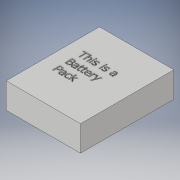
# Autodesk Inventor part: DPLX_P018_Crude_Battery_Placeholder_Smalltestmod
Saved by Autodesk Inventor 2018 (Build 220112000, 112)
## iProperties
Created: 2018-06-13
Part Number: DPLX_P018_Crude_Battery_Placeholder_Smalltestmod
Material: Generic
Document SubType Name: Modeling
Designer: DPLXuser
Density: 1 g/cm^3
Appearance: Default
Author: DPLXuser
Autodesk Inventor part; units mm, degrees
ref_plane "YZ Plane" through (0, 0, 0) normal (1, 0, 0) x (0, 1, 0)
ref_plane "XZ Plane" through (0, 0, 0) normal (0, 1, 0) x (-1, 0, 0)
ref_plane "XY Plane" through (0, 0, 0) normal (0, 0, 1) x (1, 0, 0)
sketch "Sketch1" plane through (0, 0, 0) normal (0, 1, 0) x (-1, 0, 0)
  line L0 (-30.353, 38.1) -> (30.353, 38.1)
  line L1 (30.353, 38.1) -> (30.353, -38.1)
  line L2 (30.353, -38.1) -> (-30.353, -38.1)
  line L3 (-30.353, -38.1) -> (-30.353, 38.1)
  line L4 (-30.353, 38.1) -> (30.353, -38.1) construction
  line L5 (30.353, 38.1) -> (-30.353, -38.1) construction
  point P0 (0, 0)
  dimension "d0" = 60.706
  dimension "d1" = 76.2
  constraints: 12 end point, 2 midpoint, 2 parallel, 1 horizontal, 1 perpendicular
  measures "d0" distance of L1.end L2.end
  measures "d1" distance of L0.end L1.end
extrude "Extrusion1" add sketch "Sketch1" along normal blind 20.828
sketch "Sketch2" plane through (0, 20.828, 0) normal (0, 1, 0) x (1, 0, 0)
  line L0 (-19.6689, 24.4409) -> (19.4476, 24.4409) construction
  line L1 (19.4476, 24.4409) -> (19.4476, -21.2872) construction
  line L2 (19.4476, -21.2872) -> (-19.6689, -21.2872) construction
  line L3 (-19.6689, -21.2872) -> (-19.6689, 24.4409) construction
  line L4 (-17.6287, 8.4941) -> (-17.6287, 13.8689)
  line L5 (-17.6287, 13.8689) -> (-19.6739, 13.8689)
  line L6 (-19.6739, 13.8689) -> (-19.6739, 14.5901)
  line L7 (-19.6739, 14.5901) -> (-14.7734, 14.5901)
  line L8 (-14.7734, 14.5901) -> (-14.7734, 13.8689)
  line L9 (-14.7734, 13.8689) -> (-16.8185, 13.8689)
  line L10 (-16.8185, 13.8689) -> (-16.8185, 8.4941)
  line L11 (-16.8185, 8.4941) -> (-17.6287, 8.4941)
  line L12 (-10.6237, 8.4941) -> (-11.3944, 8.4941)
  line L13 (-11.3944, 8.4941) -> (-11.3944, 11.1024)
  spline S0 degree 2 poles (-11.3944, 11.1024) (-11.3944, 11.4186) (-11.4537, 11.962) (-11.5426, 12.125) knots 0 0 0 1 2 2 2
  spline S1 degree 2 poles (-11.5426, 12.125) (-11.6364, 12.2979) (-11.9724, 12.4659) (-12.2589, 12.4659) knots 0 0 0 1 2 2 2
  spline S2 degree 2 poles (-12.2589, 12.4659) (-12.5454, 12.4659) (-13.153, 12.1596) (-13.4445, 11.9126) knots 0 0 0 1 2 2 2
  line L14 (-13.4445, 11.9126) -> (-13.4445, 8.4941)
  line L15 (-13.4445, 8.4941) -> (-14.2151, 8.4941)
  line L16 (-14.2151, 8.4941) -> (-14.2151, 14.8618)
  line L17 (-14.2151, 14.8618) -> (-13.4445, 14.8618)
  line L18 (-13.4445, 14.8618) -> (-13.4445, 12.5598)
  spline S3 degree 2 poles (-13.4445, 12.5598) (-13.0987, 12.871) (-12.4318, 13.197) (-12.0563, 13.197) knots 0 0 0 1 2 2 2
  spline S4 degree 2 poles (-12.0563, 13.197) (-11.3845, 13.197) (-10.6237, 12.3078) (-10.6237, 11.4631) knots 0 0 0 1 2 2 2
  line L19 (-10.6237, 11.4631) -> (-10.6237, 8.4941)
  line L20 (-8.7564, 8.4941) -> (-9.527, 8.4941)
  line L21 (-9.527, 8.4941) -> (-9.527, 13.0686)
  line L22 (-9.527, 13.0686) -> (-8.7564, 13.0686)
  line L23 (-8.7564, 13.0686) -> (-8.7564, 8.4941)
  line L24 (-8.7021, 13.8293) -> (-9.5764, 13.8293)
  line L25 (-9.5764, 13.8293) -> (-9.5764, 14.6296)
  line L26 (-9.5764, 14.6296) -> (-8.7021, 14.6296)
  line L27 (-8.7021, 14.6296) -> (-8.7021, 13.8293)
  spline S5 degree 2 poles (-6.3901, 8.3854) (-6.8495, 8.3854) (-7.6449, 8.6324) (-7.9067, 8.7707) knots 0 0 0 1 2 2 2
  line L28 (-7.9067, 8.7707) -> (-7.9067, 9.6353)
  line L29 (-7.9067, 9.6353) -> (-7.8672, 9.6353)
  spline S6 degree 2 poles (-7.8672, 9.6353) (-7.7684, 9.5562) (-7.5016, 9.3685) (-7.2793, 9.2648) knots 0 0 0 1 2 2 2
  spline S7 degree 2 poles (-7.2793, 9.2648) (-7.0867, 9.1709) (-6.6124, 9.0326) (-6.3605, 9.0326) knots 0 0 0 1 2 2 2
  spline S8 degree 2 poles (-6.3605, 9.0326) (-6.1777, 9.0326) (-5.7578, 9.1165) (-5.659, 9.1857) knots 0 0 0 1 2 2 2
  spline S9 degree 2 poles (-5.659, 9.1857) (-5.5157, 9.2796) (-5.3873, 9.492) (-5.3873, 9.7094) knots 0 0 0 1 2 2 2
  spline S10 degree 2 poles (-5.3873, 9.7094) (-5.3873, 9.9811) (-5.6837, 10.2626) (-6.0641, 10.3565) knots 0 0 0 1 2 2 2
  spline S11 degree 2 poles (-6.0641, 10.3565) (-6.2123, 10.3911) (-6.6865, 10.4899) (-6.8891, 10.5442) knots 0 0 0 1 2 2 2
  spline S12 degree 2 poles (-6.8891, 10.5442) (-7.4127, 10.6974) (-7.8869, 11.3297) (-7.8869, 11.7792) knots 0 0 0 1 2 2 2
  spline S13 degree 2 poles (-7.8869, 11.7792) (-7.8869, 12.4017) (-6.9533, 13.1773) (-6.1826, 13.1773) knots 0 0 0 1 2 2 2
  spline S14 degree 2 poles (-6.1826, 13.1773) (-5.8023, 13.1773) (-5.0316, 12.9895) (-4.7698, 12.8463) knots 0 0 0 1 2 2 2
  line L30 (-4.7698, 12.8463) -> (-4.7698, 12.0213)
  line L31 (-4.7698, 12.0213) -> (-4.8093, 12.0213)
  spline S15 degree 2 poles (-4.8093, 12.0213) (-5.1057, 12.2584) (-5.827, 12.5301) (-6.1975, 12.5301) knots 0 0 0 1 2 2 2
  spline S16 degree 2 poles (-6.1975, 12.5301) (-6.5778, 12.5301) (-7.1015, 12.209) (-7.1015, 11.8879) knots 0 0 0 1 2 2 2
  spline S17 degree 2 poles (-7.1015, 11.8879) (-7.1015, 11.5964) (-6.7903, 11.3149) (-6.4445, 11.2259) knots 0 0 0 1 2 2 2
  spline S18 degree 2 poles (-6.4445, 11.2259) (-6.2765, 11.1815) (-5.8517, 11.0926) (-5.6195, 11.0382) knots 0 0 0 1 2 2 2
  spline S19 degree 2 poles (-5.6195, 11.0382) (-5.1156, 10.9098) (-4.6018, 10.3219) (-4.6018, 9.8131) knots 0 0 0 1 2 2 2
  spline S20 degree 2 poles (-4.6018, 9.8131) (-4.6018, 9.5167) (-4.834, 8.993) (-5.0612, 8.8004) knots 0 0 0 1 2 2 2
  spline S21 degree 2 poles (-5.0612, 8.8004) (-5.3033, 8.5978) (-5.9208, 8.3854) (-6.3901, 8.3854) knots 0 0 0 1 2 2 2
  line L32 (-0.4818, 8.4941) -> (-1.2525, 8.4941)
  line L33 (-1.2525, 8.4941) -> (-1.2525, 13.0686)
  line L34 (-1.2525, 13.0686) -> (-0.4818, 13.0686)
  line L35 (-0.4818, 13.0686) -> (-0.4818, 8.4941)
  line L36 (-0.4275, 13.8293) -> (-1.3019, 13.8293)
  line L37 (-1.3019, 13.8293) -> (-1.3019, 14.6296)
  line L38 (-1.3019, 14.6296) -> (-0.4275, 14.6296)
  line L39 (-0.4275, 14.6296) -> (-0.4275, 13.8293)
  spline S22 degree 2 poles (1.8844, 8.3854) (1.425, 8.3854) (0.6297, 8.6324) (0.3678, 8.7707) knots 0 0 0 1 2 2 2
  line L40 (0.3678, 8.7707) -> (0.3678, 9.6353)
  line L41 (0.3678, 9.6353) -> (0.4074, 9.6353)
  spline S23 degree 2 poles (0.4074, 9.6353) (0.5062, 9.5562) (0.7729, 9.3685) (0.9952, 9.2648) knots 0 0 0 1 2 2 2
  spline S24 degree 2 poles (0.9952, 9.2648) (1.1879, 9.1709) (1.6621, 9.0326) (1.9141, 9.0326) knots 0 0 0 1 2 2 2
  spline S25 degree 2 poles (1.9141, 9.0326) (2.0969, 9.0326) (2.5168, 9.1165) (2.6156, 9.1857) knots 0 0 0 1 2 2 2
  spline S26 degree 2 poles (2.6156, 9.1857) (2.7588, 9.2796) (2.8873, 9.492) (2.8873, 9.7094) knots 0 0 0 1 2 2 2
  spline S27 degree 2 poles (2.8873, 9.7094) (2.8873, 9.9811) (2.5909, 10.2626) (2.2105, 10.3565) knots 0 0 0 1 2 2 2
  spline S28 degree 2 poles (2.2105, 10.3565) (2.0623, 10.3911) (1.588, 10.4899) (1.3855, 10.5442) knots 0 0 0 1 2 2 2
  spline S29 degree 2 poles (1.3855, 10.5442) (0.8619, 10.6974) (0.3876, 11.3297) (0.3876, 11.7792) knots 0 0 0 1 2 2 2
  spline S30 degree 2 poles (0.3876, 11.7792) (0.3876, 12.4017) (1.3213, 13.1773) (2.0919, 13.1773) knots 0 0 0 1 2 2 2
  spline S31 degree 2 poles (2.0919, 13.1773) (2.4723, 13.1773) (3.2429, 12.9895) (3.5048, 12.8463) knots 0 0 0 1 2 2 2
  line L42 (3.5048, 12.8463) -> (3.5048, 12.0213)
  line L43 (3.5048, 12.0213) -> (3.4652, 12.0213)
  spline S32 degree 2 poles (3.4652, 12.0213) (3.1688, 12.2584) (2.4476, 12.5301) (2.0771, 12.5301) knots 0 0 0 1 2 2 2
  spline S33 degree 2 poles (2.0771, 12.5301) (1.6967, 12.5301) (1.1731, 12.209) (1.1731, 11.8879) knots 0 0 0 1 2 2 2
  spline S34 degree 2 poles (1.1731, 11.8879) (1.1731, 11.5964) (1.4843, 11.3149) (1.8301, 11.2259) knots 0 0 0 1 2 2 2
  spline S35 degree 2 poles (1.8301, 11.2259) (1.9981, 11.1815) (2.4229, 11.0926) (2.6551, 11.0382) knots 0 0 0 1 2 2 2
  spline S36 degree 2 poles (2.6551, 11.0382) (3.159, 10.9098) (3.6727, 10.3219) (3.6727, 9.8131) knots 0 0 0 1 2 2 2
  spline S37 degree 2 poles (3.6727, 9.8131) (3.6727, 9.5167) (3.4405, 8.993) (3.2133, 8.8004) knots 0 0 0 1 2 2 2
  spline S38 degree 2 poles (3.2133, 8.8004) (2.9712, 8.5978) (2.3537, 8.3854) (1.8844, 8.3854) knots 0 0 0 1 2 2 2
  spline S39 degree 2 poles (9.5563, 8.9782) (9.4624, 8.9091) (9.1463, 8.6621) (8.9981, 8.588) knots 0 0 0 1 2 2 2
  spline S40 degree 2 poles (8.9981, 8.588) (8.7955, 8.4793) (8.4152, 8.3657) (8.0694, 8.3657) knots 0 0 0 1 2 2 2
  spline S41 degree 2 poles (8.0694, 8.3657) (7.7878, 8.3657) (7.279, 8.5781) (7.0863, 8.7707) knots 0 0 0 1 2 2 2
  spline S42 degree 2 poles (7.0863, 8.7707) (6.9035, 8.9585) (6.6812, 9.5118) (6.6812, 9.818) knots 0 0 0 1 2 2 2
  spline S43 degree 2 poles (6.6812, 9.818) (6.6812, 10.2923) (7.0814, 10.9641) (7.5161, 11.1568) knots 0 0 0 1 2 2 2
  spline S44 degree 2 poles (7.5161, 11.1568) (7.9014, 11.3346) (8.9487, 11.468) (9.5563, 11.5026) knots 0 0 0 1 2 2 2
  line L44 (9.5563, 11.5026) -> (9.5563, 11.6508)
  spline S45 degree 2 poles (9.5563, 11.6508) (9.5563, 11.9175) (9.3933, 12.2485) (9.2451, 12.3424) knots 0 0 0 1 2 2 2
  spline S46 degree 2 poles (9.2451, 12.3424) (9.0969, 12.4363) (8.672, 12.4955) (8.4448, 12.4955) knots 0 0 0 1 2 2 2
  spline S47 degree 2 poles (8.4448, 12.4955) (8.178, 12.4955) (7.4568, 12.3375) (7.0962, 12.1843) knots 0 0 0 1 2 2 2
  line L45 (7.0962, 12.1843) -> (7.0517, 12.1843)
  line L46 (7.0517, 12.1843) -> (7.0517, 12.9698)
  spline S48 degree 2 poles (7.0517, 12.9698) (7.2641, 13.0291) (8.0595, 13.1773) (8.4497, 13.1773) knots 0 0 0 1 2 2 2
  spline S49 degree 2 poles (8.4497, 13.1773) (8.924, 13.1773) (9.5711, 13.0291) (9.828, 12.8364) knots 0 0 0 1 2 2 2
  spline S50 degree 2 poles (9.828, 12.8364) (10.08, 12.6487) (10.327, 12.0509) (10.327, 11.6211) knots 0 0 0 1 2 2 2
  line L47 (10.327, 11.6211) -> (10.327, 8.4941)
  line L48 (10.327, 8.4941) -> (9.5563, 8.4941)
  line L49 (9.5563, 8.4941) -> (9.5563, 8.9782)
  line L50 (9.5563, 9.6204) -> (9.5563, 10.89)
  spline S51 degree 2 poles (9.5563, 10.89) (9.2797, 10.8653) (8.4448, 10.7813) (8.183, 10.7023) knots 0 0 0 1 2 2 2
  spline S52 degree 2 poles (8.183, 10.7023) (7.8767, 10.6084) (7.4766, 10.2182) (7.4766, 9.8724) knots 0 0 0 1 2 2 2
  spline S53 degree 2 poles (7.4766, 9.8724) (7.4766, 9.4772) (7.9212, 9.077) (8.346, 9.077) knots 0 0 0 1 2 2 2
  spline S54 degree 2 poles (8.346, 9.077) (8.7066, 9.077) (9.2994, 9.3883) (9.5563, 9.6204) knots 0 0 0 1 2 2 2
  spline S55 degree 2 poles (-14.9166, 0.3295) (-14.9166, -0.125) (-15.2624, -0.8216) (-15.5489, -1.0488) knots 0 0 0 1 2 2 2
  spline S56 degree 2 poles (-15.5489, -1.0488) (-15.8947, -1.3156) (-16.6802, -1.5428) (-17.3026, -1.5428) knots 0 0 0 1 2 2 2
  line L51 (-17.3026, -1.5428) -> (-19.0514, -1.5428)
  line L52 (-19.0514, -1.5428) -> (-19.0514, 4.5532)
  line L53 (-19.0514, 4.5532) -> (-17.436, 4.5532)
  spline S57 degree 2 poles (-17.436, 4.5532) (-16.7839, 4.5532) (-16.1319, 4.4692) (-15.8355, 4.3062) knots 0 0 0 1 2 2 2
  spline S58 degree 2 poles (-15.8355, 4.3062) (-15.5045, 4.1333) (-15.2031, 3.5652) (-15.2031, 3.1799) knots 0 0 0 1 2 2 2
  spline S59 degree 2 poles (-15.2031, 3.1799) (-15.2031, 2.7501) (-15.6576, 2.0684) (-16.0578, 1.8757) knots 0 0 0 1 2 2 2
  line L54 (-16.0578, 1.8757) -> (-16.0578, 1.8461)
  spline S60 degree 2 poles (-16.0578, 1.8461) (-15.5144, 1.6979) (-14.9166, 0.9124) (-14.9166, 0.3295) knots 0 0 0 1 2 2 2
  spline S61 degree 2 poles (-15.7614, 0.2949) (-15.7614, 0.6407) (-15.959, 1.0853) (-16.2554, 1.2434) knots 0 0 0 1 2 2 2
  spline S62 degree 2 poles (-16.2554, 1.2434) (-16.448, 1.3422) (-16.9025, 1.4015) (-17.3224, 1.4015) knots 0 0 0 1 2 2 2
  line L55 (-17.3224, 1.4015) -> (-18.2413, 1.4015)
  line L56 (-18.2413, 1.4015) -> (-18.2413, -0.8512)
  line L57 (-18.2413, -0.8512) -> (-17.5842, -0.8512)
  spline S63 degree 2 poles (-17.5842, -0.8512) (-17.0507, -0.8512) (-16.4381, -0.7524) (-16.201, -0.5943) knots 0 0 0 1 2 2 2
  spline S64 degree 2 poles (-16.201, -0.5943) (-15.9738, -0.4313) (-15.7614, -0.0262) (-15.7614, 0.2949) knots 0 0 0 1 2 2 2
  spline S65 degree 2 poles (-16.0479, 3.0663) (-16.0479, 3.2836) (-16.1961, 3.6097) (-16.3591, 3.7035) knots 0 0 0 1 2 2 2
  spline S66 degree 2 poles (-16.3591, 3.7035) (-16.5567, 3.8122) (-17.0359, 3.8616) (-17.4657, 3.8616) knots 0 0 0 1 2 2 2
  line L58 (-17.4657, 3.8616) -> (-18.2413, 3.8616)
  line L59 (-18.2413, 3.8616) -> (-18.2413, 2.0782)
  line L60 (-18.2413, 2.0782) -> (-17.3224, 2.0782)
  spline S67 degree 2 poles (-17.3224, 2.0782) (-16.942, 2.0782) (-16.5814, 2.1573) (-16.3887, 2.2808) knots 0 0 0 1 2 2 2
  spline S68 degree 2 poles (-16.3887, 2.2808) (-16.201, 2.3993) (-16.0479, 2.7797) (-16.0479, 3.0663) knots 0 0 0 1 2 2 2
  spline S69 degree 2 poles (-11.6216, -1.0587) (-11.7155, -1.1278) (-12.0316, -1.3748) (-12.1798, -1.4489) knots 0 0 0 1 2 2 2
  spline S70 degree 2 poles (-12.1798, -1.4489) (-12.3824, -1.5576) (-12.7628, -1.6712) (-13.1086, -1.6712) knots 0 0 0 1 2 2 2
  spline S71 degree 2 poles (-13.1086, -1.6712) (-13.3901, -1.6712) (-13.899, -1.4588) (-14.0916, -1.2662) knots 0 0 0 1 2 2 2
  spline S72 degree 2 poles (-14.0916, -1.2662) (-14.2744, -1.0784) (-14.4967, -0.5252) (-14.4967, -0.2189) knots 0 0 0 1 2 2 2
  spline S73 degree 2 poles (-14.4967, -0.2189) (-14.4967, 0.2554) (-14.0966, 0.9272) (-13.6618, 1.1199) knots 0 0 0 1 2 2 2
  spline S74 degree 2 poles (-13.6618, 1.1199) (-13.2765, 1.2977) (-12.2292, 1.4311) (-11.6216, 1.4657) knots 0 0 0 1 2 2 2
  line L61 (-11.6216, 1.4657) -> (-11.6216, 1.6139)
  spline S75 degree 2 poles (-11.6216, 1.6139) (-11.6216, 1.8806) (-11.7846, 2.2116) (-11.9328, 2.3055) knots 0 0 0 1 2 2 2
  spline S76 degree 2 poles (-11.9328, 2.3055) (-12.081, 2.3993) (-12.5059, 2.4586) (-12.7331, 2.4586) knots 0 0 0 1 2 2 2
  spline S77 degree 2 poles (-12.7331, 2.4586) (-12.9999, 2.4586) (-13.7211, 2.3005) (-14.0817, 2.1474) knots 0 0 0 1 2 2 2
  line L62 (-14.0817, 2.1474) -> (-14.1262, 2.1474)
  line L63 (-14.1262, 2.1474) -> (-14.1262, 2.9329)
  spline S78 degree 2 poles (-14.1262, 2.9329) (-13.9138, 2.9922) (-13.1184, 3.1404) (-12.7282, 3.1404) knots 0 0 0 1 2 2 2
  spline S79 degree 2 poles (-12.7282, 3.1404) (-12.2539, 3.1404) (-11.6068, 2.9922) (-11.3499, 2.7995) knots 0 0 0 1 2 2 2
  spline S80 degree 2 poles (-11.3499, 2.7995) (-11.098, 2.6118) (-10.851, 2.014) (-10.851, 1.5842) knots 0 0 0 1 2 2 2
  line L64 (-10.851, 1.5842) -> (-10.851, -1.5428)
  line L65 (-10.851, -1.5428) -> (-11.6216, -1.5428)
  line L66 (-11.6216, -1.5428) -> (-11.6216, -1.0587)
  line L67 (-11.6216, -0.4165) -> (-11.6216, 0.8531)
  spline S81 degree 2 poles (-11.6216, 0.8531) (-11.8983, 0.8284) (-12.7331, 0.7444) (-12.9949, 0.6654) knots 0 0 0 1 2 2 2
  spline S82 degree 2 poles (-12.9949, 0.6654) (-13.3012, 0.5715) (-13.7014, 0.1813) (-13.7014, -0.1645) knots 0 0 0 1 2 2 2
  spline S83 degree 2 poles (-13.7014, -0.1645) (-13.7014, -0.5597) (-13.2568, -0.9599) (-12.8319, -0.9599) knots 0 0 0 1 2 2 2
  spline S84 degree 2 poles (-12.8319, -0.9599) (-12.4713, -0.9599) (-11.8785, -0.6487) (-11.6216, -0.4165) knots 0 0 0 1 2 2 2
  spline S85 degree 2 poles (-8.3859, -1.6317) (-9.0133, -1.6317) (-9.7197, -0.9154) (-9.7197, -0.1398) knots 0 0 0 1 2 2 2
  line L68 (-9.7197, -0.1398) -> (-9.7197, 2.3944)
  line L69 (-9.7197, 2.3944) -> (-10.2384, 2.3944)
  line L70 (-10.2384, 2.3944) -> (-10.2384, 3.0317)
  line L71 (-10.2384, 3.0317) -> (-9.7197, 3.0317)
  line L72 (-9.7197, 3.0317) -> (-9.7197, 4.3457)
  line L73 (-9.7197, 4.3457) -> (-8.9491, 4.3457)
  line L74 (-8.9491, 4.3457) -> (-8.9491, 3.0317)
  line L75 (-8.9491, 3.0317) -> (-7.5313, 3.0317)
  line L76 (-7.5313, 3.0317) -> (-7.5313, 2.3944)
  line L77 (-7.5313, 2.3944) -> (-8.9491, 2.3944)
  line L78 (-8.9491, 2.3944) -> (-8.9491, 0.2159)
  spline S86 degree 2 poles (-8.9491, 0.2159) (-8.9491, -0.1299) (-8.9244, -0.5103) (-8.8404, -0.6734) knots 0 0 0 1 2 2 2
  spline S87 degree 2 poles (-8.8404, -0.6734) (-8.7712, -0.8166) (-8.46, -0.9599) (-8.1932, -0.9599) knots 0 0 0 1 2 2 2
  spline S88 degree 2 poles (-8.1932, -0.9599) (-8.0055, -0.9599) (-7.6548, -0.8463) (-7.5757, -0.8117) knots 0 0 0 1 2 2 2
  line L79 (-7.5757, -0.8117) -> (-7.5313, -0.8117)
  line L80 (-7.5313, -0.8117) -> (-7.5313, -1.5033)
  spline S89 degree 2 poles (-7.5313, -1.5033) (-7.7486, -1.5626) (-8.1932, -1.6317) (-8.3859, -1.6317) knots 0 0 0 1 2 2 2
  spline S90 degree 2 poles (-5.58, -1.6317) (-6.2073, -1.6317) (-6.9138, -0.9154) (-6.9138, -0.1398) knots 0 0 0 1 2 2 2
  line L81 (-6.9138, -0.1398) -> (-6.9138, 2.3944)
  line L82 (-6.9138, 2.3944) -> (-7.4325, 2.3944)
  line L83 (-7.4325, 2.3944) -> (-7.4325, 3.0317)
  line L84 (-7.4325, 3.0317) -> (-6.9138, 3.0317)
  line L85 (-6.9138, 3.0317) -> (-6.9138, 4.3457)
  line L86 (-6.9138, 4.3457) -> (-6.1431, 4.3457)
  line L87 (-6.1431, 4.3457) -> (-6.1431, 3.0317)
  line L88 (-6.1431, 3.0317) -> (-4.7253, 3.0317)
  line L89 (-4.7253, 3.0317) -> (-4.7253, 2.3944)
  line L90 (-4.7253, 2.3944) -> (-6.1431, 2.3944)
  line L91 (-6.1431, 2.3944) -> (-6.1431, 0.2159)
  spline S91 degree 2 poles (-6.1431, 0.2159) (-6.1431, -0.1299) (-6.1184, -0.5103) (-6.0344, -0.6734) knots 0 0 0 1 2 2 2
  spline S92 degree 2 poles (-6.0344, -0.6734) (-5.9653, -0.8166) (-5.6541, -0.9599) (-5.3873, -0.9599) knots 0 0 0 1 2 2 2
  spline S93 degree 2 poles (-5.3873, -0.9599) (-5.1996, -0.9599) (-4.8488, -0.8463) (-4.7698, -0.8117) knots 0 0 0 1 2 2 2
  line L92 (-4.7698, -0.8117) -> (-4.7253, -0.8117)
  line L93 (-4.7253, -0.8117) -> (-4.7253, -1.5033)
  spline S94 degree 2 poles (-4.7253, -1.5033) (-4.9427, -1.5626) (-5.3873, -1.6317) (-5.58, -1.6317) knots 0 0 0 1 2 2 2
  spline S95 degree 2 poles (-2.1713, -1.6465) (-3.268, -1.6465) (-4.4734, -0.4165) (-4.4734, 0.7197) knots 0 0 0 1 2 2 2
  spline S96 degree 2 poles (-4.4734, 0.7197) (-4.4734, 1.8362) (-3.3026, 3.1601) (-2.3591, 3.1601) knots 0 0 0 1 2 2 2
  spline S97 degree 2 poles (-2.3591, 3.1601) (-1.9342, 3.1601) (-1.2772, 2.9131) (-1.0351, 2.6513) knots 0 0 0 1 2 2 2
  spline S98 degree 2 poles (-1.0351, 2.6513) (-0.7881, 2.3895) (-0.5263, 1.6336) (-0.5263, 1.0853) knots 0 0 0 1 2 2 2
  line L94 (-0.5263, 1.0853) -> (-0.5263, 0.6654)
  line L95 (-0.5263, 0.6654) -> (-3.6929, 0.6654)
  spline S99 degree 2 poles (-3.6929, 0.6654) (-3.6929, -0.1299) (-2.8926, -0.9747) (-2.1812, -0.9747) knots 0 0 0 1 2 2 2
  spline S100 degree 2 poles (-2.1812, -0.9747) (-1.9293, -0.9747) (-1.4402, -0.8611) (-1.2426, -0.7722) knots 0 0 0 1 2 2 2
  spline S101 degree 2 poles (-1.2426, -0.7722) (-1.0351, -0.6734) (-0.7486, -0.5005) (-0.6547, -0.4214) knots 0 0 0 1 2 2 2
  line L96 (-0.6547, -0.4214) -> (-0.6103, -0.4214)
  line L97 (-0.6103, -0.4214) -> (-0.6103, -1.2612)
  spline S102 degree 2 poles (-0.6103, -1.2612) (-0.7437, -1.3156) (-1.1487, -1.4736) (-1.3068, -1.5181) knots 0 0 0 1 2 2 2
  spline S103 degree 2 poles (-1.3068, -1.5181) (-1.5291, -1.5823) (-1.8947, -1.6465) (-2.1713, -1.6465) knots 0 0 0 1 2 2 2
  spline S104 degree 2 poles (-1.2772, 1.2533) (-1.2871, 1.5645) (-1.4155, 2.019) (-1.539, 2.1721) knots 0 0 0 1 2 2 2
  spline S105 degree 2 poles (-1.539, 2.1721) (-1.6724, 2.345) (-2.0923, 2.5278) (-2.4035, 2.5278) knots 0 0 0 1 2 2 2
  spline S106 degree 2 poles (-2.4035, 2.5278) (-2.7098, 2.5278) (-3.1396, 2.345) (-3.3174, 2.1672) knots 0 0 0 1 2 2 2
  spline S107 degree 2 poles (-3.3174, 2.1672) (-3.4903, 1.9844) (-3.6682, 1.5447) (-3.6929, 1.2533) knots 0 0 0 1 2 2 2
  line L98 (-3.6929, 1.2533) -> (-1.2772, 1.2533)
  line L99 (2.6798, 2.2067) -> (2.6403, 2.2067)
  spline S108 degree 2 poles (2.6403, 2.2067) (2.5513, 2.2314) (2.3587, 2.2413) (2.2253, 2.2413) knots 0 0 0 1 2 2 2
  spline S109 degree 2 poles (2.2253, 2.2413) (1.9141, 2.2413) (1.3015, 1.9696) (1.0249, 1.7028) knots 0 0 0 1 2 2 2
  line L100 (1.0249, 1.7028) -> (1.0249, -1.5428)
  line L101 (1.0249, -1.5428) -> (0.2542, -1.5428)
  line L102 (0.2542, -1.5428) -> (0.2542, 3.0317)
  line L103 (0.2542, 3.0317) -> (1.0249, 3.0317)
  line L104 (1.0249, 3.0317) -> (1.0249, 2.3499)
  spline S110 degree 2 poles (1.0249, 2.3499) (1.4448, 2.7254) (2.0722, 3.0317) (2.3686, 3.0317) knots 0 0 0 1 2 2 2
  spline S111 degree 2 poles (2.3686, 3.0317) (2.4871, 3.0317) (2.6057, 3.0218) (2.6798, 3.007) knots 0 0 0 1 2 2 2
  line L105 (2.6798, 3.007) -> (2.6798, 2.2067)
  line L106 (6.8689, 3.0317) -> (4.4088, -3.2273)
  line L107 (4.4088, -3.2273) -> (3.5838, -3.2273)
  line L108 (3.5838, -3.2273) -> (4.4039, -1.3205)
  line L109 (4.4039, -1.3205) -> (2.744, 3.0317)
  line L110 (2.744, 3.0317) -> (3.5739, 3.0317)
  line L111 (3.5739, 3.0317) -> (4.8238, -0.3572)
  line L112 (4.8238, -0.3572) -> (6.0686, 3.0317)
  line L113 (6.0686, 3.0317) -> (6.8689, 3.0317)
  spline S112 degree 2 poles (-15.1982, -7.3214) (-15.1982, -7.7166) (-15.4798, -8.428) (-15.7317, -8.675) knots 0 0 0 1 2 2 2
  spline S113 degree 2 poles (-15.7317, -8.675) (-16.0479, -8.9862) (-16.9025, -9.3073) (-17.5546, -9.3073) knots 0 0 0 1 2 2 2
  line L114 (-17.5546, -9.3073) -> (-18.2413, -9.3073)
  line L115 (-18.2413, -9.3073) -> (-18.2413, -11.5797)
  line L116 (-18.2413, -11.5797) -> (-19.0514, -11.5797)
  line L117 (-19.0514, -11.5797) -> (-19.0514, -5.4837)
  line L118 (-19.0514, -5.4837) -> (-17.52, -5.4837)
  spline S114 degree 2 poles (-17.52, -5.4837) (-16.9766, -5.4837) (-16.2158, -5.6615) (-15.9244, -5.8641) knots 0 0 0 1 2 2 2
  spline S115 degree 2 poles (-15.9244, -5.8641) (-15.5835, -6.0963) (-15.1982, -6.8126) (-15.1982, -7.3214) knots 0 0 0 1 2 2 2
  spline S116 degree 2 poles (-16.0429, -7.3461) (-16.0429, -7.0299) (-16.2603, -6.5656) (-16.4826, -6.4174) knots 0 0 0 1 2 2 2
  spline S117 degree 2 poles (-16.4826, -6.4174) (-16.6753, -6.2889) (-17.189, -6.1852) (-17.5694, -6.1852) knots 0 0 0 1 2 2 2
  line L119 (-17.5694, -6.1852) -> (-18.2413, -6.1852)
  line L120 (-18.2413, -6.1852) -> (-18.2413, -8.6157)
  line L121 (-18.2413, -8.6157) -> (-17.688, -8.6157)
  spline S118 degree 2 poles (-17.688, -8.6157) (-17.194, -8.6157) (-16.5863, -8.4576) (-16.3887, -8.2501) knots 0 0 0 1 2 2 2
  spline S119 degree 2 poles (-16.3887, -8.2501) (-16.206, -8.0673) (-16.0429, -7.6376) (-16.0429, -7.3461) knots 0 0 0 1 2 2 2
  spline S120 degree 2 poles (-11.9378, -11.0956) (-12.0316, -11.1647) (-12.3478, -11.4117) (-12.496, -11.4858) knots 0 0 0 1 2 2 2
  spline S121 degree 2 poles (-12.496, -11.4858) (-12.6985, -11.5945) (-13.0789, -11.7081) (-13.4247, -11.7081) knots 0 0 0 1 2 2 2
  spline S122 degree 2 poles (-13.4247, -11.7081) (-13.7063, -11.7081) (-14.2151, -11.4957) (-14.4078, -11.3031) knots 0 0 0 1 2 2 2
  spline S123 degree 2 poles (-14.4078, -11.3031) (-14.5906, -11.1153) (-14.8129, -10.5621) (-14.8129, -10.2558) knots 0 0 0 1 2 2 2
  spline S124 degree 2 poles (-14.8129, -10.2558) (-14.8129, -9.7815) (-14.4127, -9.1097) (-13.978, -8.917) knots 0 0 0 1 2 2 2
  spline S125 degree 2 poles (-13.978, -8.917) (-13.5927, -8.7392) (-12.5454, -8.6058) (-11.9378, -8.5712) knots 0 0 0 1 2 2 2
  line L122 (-11.9378, -8.5712) -> (-11.9378, -8.423)
  spline S126 degree 2 poles (-11.9378, -8.423) (-11.9378, -8.1563) (-12.1008, -7.8253) (-12.249, -7.7314) knots 0 0 0 1 2 2 2
  spline S127 degree 2 poles (-12.249, -7.7314) (-12.3972, -7.6376) (-12.822, -7.5783) (-13.0493, -7.5783) knots 0 0 0 1 2 2 2
  spline S128 degree 2 poles (-13.0493, -7.5783) (-13.316, -7.5783) (-14.0373, -7.7364) (-14.3979, -7.8895) knots 0 0 0 1 2 2 2
  line L123 (-14.3979, -7.8895) -> (-14.4424, -7.8895)
  line L124 (-14.4424, -7.8895) -> (-14.4424, -7.104)
  spline S129 degree 2 poles (-14.4424, -7.104) (-14.2299, -7.0448) (-13.4346, -6.8966) (-13.0443, -6.8966) knots 0 0 0 1 2 2 2
  spline S130 degree 2 poles (-13.0443, -6.8966) (-12.5701, -6.8966) (-11.923, -7.0448) (-11.6661, -7.2374) knots 0 0 0 1 2 2 2
  spline S131 degree 2 poles (-11.6661, -7.2374) (-11.4141, -7.4251) (-11.1671, -8.0229) (-11.1671, -8.4527) knots 0 0 0 1 2 2 2
  line L125 (-11.1671, -8.4527) -> (-11.1671, -11.5797)
  line L126 (-11.1671, -11.5797) -> (-11.9378, -11.5797)
  line L127 (-11.9378, -11.5797) -> (-11.9378, -11.0956)
  line L128 (-11.9378, -10.4534) -> (-11.9378, -9.1838)
  spline S132 degree 2 poles (-11.9378, -9.1838) (-12.2144, -9.2085) (-13.0493, -9.2925) (-13.3111, -9.3715) knots 0 0 0 1 2 2 2
  spline S133 degree 2 poles (-13.3111, -9.3715) (-13.6174, -9.4654) (-14.0175, -9.8556) (-14.0175, -10.2014) knots 0 0 0 1 2 2 2
  spline S134 degree 2 poles (-14.0175, -10.2014) (-14.0175, -10.5966) (-13.5729, -10.9968) (-13.1481, -10.9968) knots 0 0 0 1 2 2 2
  spline S135 degree 2 poles (-13.1481, -10.9968) (-12.7875, -10.9968) (-12.1947, -10.6856) (-11.9378, -10.4534) knots 0 0 0 1 2 2 2
  spline S136 degree 2 poles (-8.2673, -11.6834) (-8.7416, -11.6834) (-9.527, -11.392) (-9.8086, -11.0956) knots 0 0 0 1 2 2 2
  spline S137 degree 2 poles (-9.8086, -11.0956) (-10.0902, -10.8041) (-10.4014, -9.905) (-10.4014, -9.3023) knots 0 0 0 1 2 2 2
  spline S138 degree 2 poles (-10.4014, -9.3023) (-10.4014, -8.6997) (-10.0803, -7.8203) (-9.8086, -7.5239) knots 0 0 0 1 2 2 2
  spline S139 degree 2 poles (-9.8086, -7.5239) (-9.5369, -7.2226) (-8.7317, -6.9015) (-8.2673, -6.9015) knots 0 0 0 1 2 2 2
  spline S140 degree 2 poles (-8.2673, -6.9015) (-7.8919, -6.9015) (-7.1904, -7.1139) (-6.9187, -7.2522) knots 0 0 0 1 2 2 2
  line L129 (-6.9187, -7.2522) -> (-6.9187, -8.1167)
  line L130 (-6.9187, -8.1167) -> (-6.9632, -8.1167)
  spline S141 degree 2 poles (-6.9632, -8.1167) (-7.0471, -8.0476) (-7.304, -7.8697) (-7.4868, -7.7759) knots 0 0 0 1 2 2 2
  spline S142 degree 2 poles (-7.4868, -7.7759) (-7.6498, -7.6968) (-8.0845, -7.5733) (-8.2821, -7.5733) knots 0 0 0 1 2 2 2
  spline S143 degree 2 poles (-8.2821, -7.5733) (-8.8799, -7.5733) (-9.6061, -8.4774) (-9.6061, -9.3023) knots 0 0 0 1 2 2 2
  spline S144 degree 2 poles (-9.6061, -9.3023) (-9.6061, -10.1076) (-8.9046, -11.0116) (-8.2821, -11.0116) knots 0 0 0 1 2 2 2
  spline S145 degree 2 poles (-8.2821, -11.0116) (-7.9067, -11.0116) (-7.225, -10.7004) (-6.9632, -10.4583) knots 0 0 0 1 2 2 2
  line L131 (-6.9632, -10.4583) -> (-6.9187, -10.4583)
  line L132 (-6.9187, -10.4583) -> (-6.9187, -11.3228)
  spline S146 degree 2 poles (-6.9187, -11.3228) (-7.0323, -11.3772) (-7.3781, -11.5303) (-7.5164, -11.5649) knots 0 0 0 1 2 2 2
  spline S147 degree 2 poles (-7.5164, -11.5649) (-7.714, -11.6242) (-8.0253, -11.6834) (-8.2673, -11.6834) knots 0 0 0 1 2 2 2
  line L133 (-2.4282, -11.5797) -> (-3.4409, -11.5797)
  line L134 (-3.4409, -11.5797) -> (-5.1403, -9.3715)
  line L135 (-5.1403, -9.3715) -> (-5.4466, -9.6679)
  line L136 (-5.4466, -9.6679) -> (-5.4466, -11.5797)
  line L137 (-5.4466, -11.5797) -> (-6.2172, -11.5797)
  line L138 (-6.2172, -11.5797) -> (-6.2172, -5.212)
  line L139 (-6.2172, -5.212) -> (-5.4466, -5.212)
  line L140 (-5.4466, -5.212) -> (-5.4466, -8.9368)
  line L141 (-5.4466, -8.9368) -> (-3.6385, -7.0052)
  line L142 (-3.6385, -7.0052) -> (-2.6802, -7.0052)
  line L143 (-2.6802, -7.0052) -> (-4.5574, -8.917)
  line L144 (-4.5574, -8.917) -> (-2.4282, -11.5797)
  point P0 (0, 0)
  constraints: 2 other
emboss "Emboss1" sketch "Sketch2" operation cut depth 2.54 direction (0, -1, 0)
body "Solid1"
